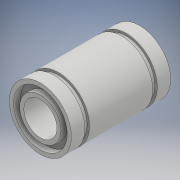
# Autodesk Inventor part: rolamento_linear_lm8uu.iam
Saved by Autodesk Inventor 2018 (Build 220112000, 112)
## iProperties
Created: 2018-05-16
Part Number: rolamento_linear_lm8uu.iam
Material: Genérico
Document SubType Name: Modeling
Designer: Usuario
Density: 1 g/cm^3
Appearance: Padrão
Mass: 6.471 g
Surface Area: 72.2059 cm^2
Volume: 6.471 cm^3
Author: Usuario
Autodesk Inventor part; units mm, degrees
ref_plane "YZ Plane" through (0, 0, 0) normal (1, 0, 0) x (0, 1, 0)
ref_plane "XZ Plane" through (0, 0, 0) normal (0, 1, 0) x (-1, 0, 0)
ref_plane "XY Plane" through (0, 0, 0) normal (0, 0, 1) x (1, 0, 0)
sketch "Esboço1" plane through (0, 0, 0) normal (0, 0, 1) x (1, 0, 0)
  line L0 (-7.5, 0) -> (-7.5, 3.25)
  line L1 (-7.5, 3.25) -> (-6.95, 3.25)
  line L2 (-6.95, 3.25) -> (-6.95, 4.35)
  line L3 (-6.95, 4.35) -> (-7.5, 4.35)
  line L4 (-7.5, 4.35) -> (-7.5, 19.65)
  line L5 (-7.5, 19.65) -> (-6.95, 19.65)
  line L6 (-6.95, 19.65) -> (-6.95, 20.75)
  line L7 (-6.95, 20.75) -> (-7.5, 20.75)
  line L8 (-7.5, 20.75) -> (-7.5, 24)
  line L9 (-7.5, 24) -> (-6.5, 24)
  line L10 (-7.5, 0) -> (-6.5, 0)
  line L11 (-6.5, 0) -> (0, 0) construction
  line L12 (0, 0) -> (0, 24) construction
  line L13 (0, 24) -> (-6.5, 24) construction
  line L14 (-6.5, 24) -> (-6.5, 0)
  dimension "d0" = 6.5
  dimension "d1" = 24
  dimension "d4" = 0.55
  dimension "d5" = 1.1
  dimension "d6" = 1.1
  dimension "d8" = 1
  dimension "d26" = 17.5
  dimension "d27" = 3.25
  constraints: 30 end point, 10 perpendicular, 6 point on line, 2 horizontal
  measures "d0" distance of L12.end L9.end
  measures "d1" distance of L0.start L8.end
  measures "d4" distance between parallel lines of L6 L4
  measures "d5" distance of L5.end L6.end
  measures "d6" distance of L1.end L2.end
  measures "d8" distance of L8.end L9.end
  measures "d26" distance between parallel lines of L1 L7
  measures "d27" distance of L0.start L0.end
sketch "Esboço3" plane through (0, 0, 0) normal (0, 0, 1) x (1, 0, 0)
  line L0 (0, 24) -> (0, 0) construction
  line L1 (0, 24) -> (0, 35.5) construction
  line L2 (0, 0) -> (0, 1.5) construction
  line L3 (-4, 0) -> (-4, 24)
  line L4 (-4, 0) -> (-5, 0)
  line L5 (-5, 24) -> (-4, 24)
  line L6 (-5, 1.5) -> (-6.4, 1.5)
  line L7 (-6.4, 1.5) -> (-6.4, 22.5)
  line L8 (-6.4, 22.5) -> (-5, 22.5)
  line L9 (-5, 0) -> (-5, 1.5)
  line L10 (-5, 22.5) -> (-5, 24)
  dimension "d28" = 24
  dimension "d30" = 4
  dimension "d31" = 21
  dimension "d32" = 24
  dimension "d33" = 1.5
  dimension "d34" = 2.4
  dimension "d36" = 1
  dimension "d37" = 1
  constraints: 22 end point, 5 perpendicular, 2 horizontal, 2 point on line, 1 parallel, 1 vertical
  measures "d28" distance of L0.start L0.end
  measures "d30" distance between parallel lines of L3 L0
  measures "d31" distance of L6.end L7.end
  measures "d32" distance of L3.start L3.end
  measures "d33" distance of L4.end L6.start
  measures "d34" distance between parallel lines of L7 L3
  measures "d36" distance of L3.start L4.end
  measures "d37" distance of L5.start L3.end
revolve "Revolução1" add sketch "Esboço3" angle 360 about axis through (0, 24, 0) along (0, -1, 0)
revolve "Revolução2" add sketch "Esboço1" angle 360 about axis through (0, 0, 0) along (0, 1, 0)
equation "\"d6\" = d5"
equation "\"d27\" = -0.5 * d26 + 0.5 * d1"
equation "\"d33\" = -0.5 * d31 + 0.5 * d32"
equation "\"d37\" = d36"
